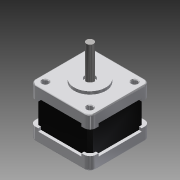
# Autodesk Inventor part: NEMA 17 Stepper
Saved by Autodesk Inventor 2015 (Build 190159000, 159)
## iProperties
Created: 2015-02-20
Part Number: NEMA 17 Stepper
Material: Generic
Document SubType Name: Modeling
Designer: pltwe4
Density: 1 g/cm^3
Appearance: Aluminum - Polished
Author: pltwe4
Autodesk Inventor part; units mm, degrees
ref_plane "YZ Plane" through (0, 0, 0) normal (1, 0, 0) x (0, 1, 0)
ref_plane "XZ Plane" through (0, 0, 0) normal (0, 1, 0) x (-1, 0, 0)
ref_plane "XY Plane" through (0, 0, 0) normal (0, 0, 1) x (1, 0, 0)
sketch "Sketch1" plane through (0, 0, 0) normal (0, 1, 0) x (-1, 0, 0)
  line L0 (17, 21) -> (-17, 21)
  line L1 (-21, 17) -> (-21, -17)
  line L2 (-17, -21) -> (17, -21)
  line L3 (21, -17) -> (21, 17)
  line L4 (0, -30.5598) -> (0, 30.5598) projected
  line L5 (-30.5598, 0) -> (30.5598, 0) projected
  circle A0 centre (0, 0) radius 2.5
  circle A1 centre (0, 0) radius 3.5
  circle A2 centre (0, 0) radius 11
  circle A3 centre (15.5, 15.5) radius 2
  circle A4 centre (15.5, -15.5) radius 2
  circle A5 centre (-15.5, -15.5) radius 2
  circle A6 centre (-15.5, 15.5) radius 2
  arc A7 (21, 17) -> (17, 21) centre (17, 17) ccw
  arc A8 (17, -21) -> (21, -17) centre (17, -17) ccw
  arc A9 (-21, -17) -> (-17, -21) centre (-17, -17) ccw
  arc A10 (-17, 21) -> (-21, 17) centre (-17, 17) ccw
  point P0 (21, 21)
  point P1 (21, -21)
  dimension "d0" = 5
  dimension "d1" = 7
  dimension "d2" = 22
  dimension "d3" = 42
  dimension "d4" = 4
  dimension "d5" = 31
  dimension "d6" = 31
  dimension "d7" = 4
  constraints: 11 centre point, 8 end point, 8 point on circle, 8 tangent, 4 point on line, 3 coincident, 3 equal radius, 2 parallel, 2 perpendicular, 1 horizontal, 5 other
  measures "d0" diameter of A0
  measures "d1" diameter of A1
  measures "d2" diameter of A2
  measures "d3" distance of point (21, -21) point (21, 21)
  measures "d4" diameter of A3
  measures "d5" distance of A4.centre A3.centre
  measures "d6" distance of A6.centre A3.centre
  measures "d7" radius of A7
extrude "Extrusion1" add sketch "Sketch1" against normal blind 34 contours A7 L3 L5 A2 L4 L0 | L4 A2 L5 L1 A10 L0 | A2 L5 A1 L4 | L4 A1 L5 A2 | L3 A8 L2 L4 A2 L5 | A1 L5 A0 L4 | L4 A0 L5 A1 | A2 L4 A1 L5 | A2 L4 L2 A9 L1 L5 | L5 A1 L4 A2 | A1 L4 A0 L5 | L5 A0 L4 A1
extrude "Extrusion2" add sketch "Sketch1" along normal blind 2 contours A2 L5 A1 L4 | L4 A1 L5 A2 | A2 L4 A1 L5 | L5 A1 L4 A2
sketch "Sketch2" plane through (21, 0, 17) normal (1, 0, 0) x (0, 0, -1)
  line L0 (-4, 0) -> (0, 0) projected
  line L1 (0, -34) -> (-4, -34) projected
  line L2 (0, 0) -> (34, 0) projected
  line L3 (34, -34) -> (0, -34) projected
  line L4 (34, 0) -> (38, 0) projected
  line L5 (38, -34) -> (34, -34) projected
  line L6 (-4, -9) -> (2, -9)
  line L7 (2, -9) -> (2, -7)
  line L8 (2, -7) -> (32, -7)
  line L9 (32, -7) -> (32, -9)
  line L10 (32, -9) -> (38, -9)
  line L11 (-4, 0) -> (-4, -34) projected
  line L12 (-4, -25) -> (2, -25)
  line L13 (2, -25) -> (2, -27)
  line L14 (2, -27) -> (32, -27)
  line L15 (32, -27) -> (32, -25)
  line L16 (32, -25) -> (38, -25)
  line L17 (38, 0) -> (38, -34) projected
  line L18 (-4, -17) -> (38, -17) construction
  line L19 (-4, 0) -> (-4, -9)
  line L20 (-4, -25) -> (-4, -34)
  line L21 (38, 0) -> (38, -9)
  line L22 (38, -25) -> (38, -34)
  line L23 (17, -41.2) -> (17, 9.2) construction
  line L24 (-4, -9) -> (-4, -25)
  line L25 (38, -25) -> (38, -9)
  point P0 (17, 0)
  dimension "d12" = 6
  dimension "d13" = 7
  dimension "d14" = 2
  constraints: 34 end point, 9 point on line, 5 perpendicular, 2 collinear, 2 horizontal, 2 midpoint, 2 parallel, 5 other
  measures "d12" distance between parallel lines of L11 L7
  measures "d13" distance between parallel lines of L2 L8
  measures "d14" distance between parallel lines of L8 L6
extrude "Extrusion3" cut sketch "Sketch2" against normal blind 2 contours L6 L7 L8 L9 L10 L17 L16 L15 L14 L13 L12 L11
pattern_circular "Circular Pattern1" count 4 over 360 about axis through (0, 0, 0) along (0, -1, 0) of "Extrusion3"
chamfer "Chamfer1" distance 2 angle 45 4 edges at (-19, -17, 19) (-19, -17, -19) (19, -17, 19) (19, -17, -19)
sketch "Sketch3" plane through (0, -34, 0) normal (0, -1, 0) x (1, 0, 0)
  circle A0 centre (0, 0) radius 2.5 projected
  circle A1 centre (15.5, 15.5) radius 2 projected
  circle A2 centre (15.5, -15.5) radius 2 projected
  circle A3 centre (-15.5, -15.5) radius 2 projected
  circle A4 centre (-15.5, 15.5) radius 2 projected
  line L0 (17, 21) -> (-17, 21) projected
  arc A5 (-17, 21) -> (-21, 17) centre (-17, 17) ccw projected
  line L1 (-21, 17) -> (-21, -17) projected
  arc A6 (-21, -17) -> (-17, -21) centre (-17, -17) ccw projected
  line L2 (-17, -21) -> (17, -21) projected
  arc A7 (17, -21) -> (21, -17) centre (17, -17) ccw projected
  line L3 (21, -17) -> (21, 17) projected
  arc A8 (21, 17) -> (17, 21) centre (17, 17) ccw projected
extrude "Extrusion4" add sketch "Sketch3" against normal blind 58 contours A0
chamfer "Chamfer2" distance 0.5 angle 45 4 edges at (-13.5, 0, -15.5) (-13.5, 0, 15.5) (17.5, 0, 15.5) (17.5, 0, -15.5)
fillet "Fillet1" radius 1 16 edges at (-19.8284, 0, -19.8284) (-21, 0, 0) (-19.8284, 0, 19.8284) (0, 0, 21) (19.8284, 0, 19.8284) (21, 0, 0) (19.8284, 0, -19.8284) (0, 0, -21) (19.8284, -34, 19.8284) (0, -34, 21) (-19.8284, -34, 19.8284) (-21, -34, 0) (-19.8284, -34, -19.8284) (0, -34, -21) (19.8284, -34, -19.8284) (21, -34, 0)
body "Solid1"
